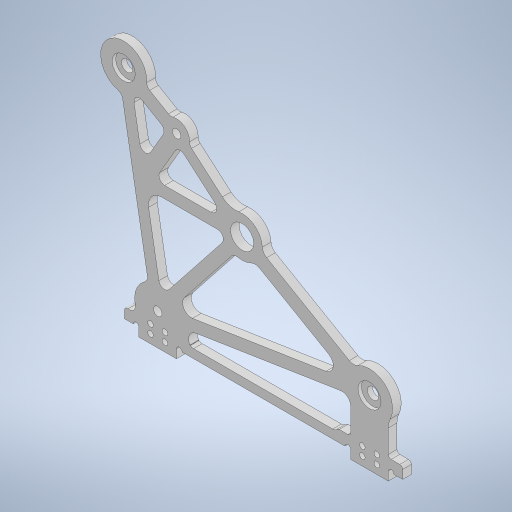
# Autodesk Inventor part: 左フレーム
Saved by Autodesk Inventor 2023 (Build 270158000, 158)
## iProperties
Created: 2022-05-09
Part Number: 左フレーム
Material: 一般
Document SubType Name: Modeling
Designer: muzho
Density: 1 g/cm^3
Appearance: 既定
Author: muzho
Autodesk Inventor part; units mm, degrees
ref_plane "YZ Plane" through (0, 0, 0) normal (1, 0, 0) x (0, 1, 0)
ref_plane "XZ Plane" through (0, 0, 0) normal (0, 1, 0) x (-1, 0, 0)
ref_plane "XY Plane" through (0, 0, 0) normal (0, 0, 1) x (1, 0, 0)
sketch "スケッチ1" plane through (0, 0, 0) normal (0, 0, 1) x (1, 0, 0)
  circle A0 centre (96.1264, 13.4764) radius 8
  circle A1 centre (96.1264, 13.4764) radius 4
  circle A2 centre (11.0035, 69.2097) radius 8
  circle A3 centre (52, 38.9528) radius 37.9528 construction
  circle A4 centre (22.7682, 2) radius 1.5
  circle A5 centre (112.1264, -3) radius 3
  circle A6 centre (112.1264, -3) radius 1.5
  circle A7 centre (74.5, -6) radius 1
  circle A8 centre (69.5, -6) radius 1
  circle A9 centre (69.5, -3) radius 1
  circle A10 centre (74.5, -3) radius 1
  circle A11 centre (64.5, -6) radius 1
  circle A12 centre (79.5, -6) radius 1
  line L0 (65.5, -6) -> (65.5, -9)
  line L1 (65.5, -9) -> (72, -9)
  line L2 (78.5, -9) -> (72, -9)
  line L3 (78.5, -6) -> (78.5, -9)
  circle A13 centre (-14.8489, -6) radius 1
  line L4 (-13.8489, -6) -> (-13.8489, -9)
  line L5 (-13.8489, -9) -> (-7.3489, -9)
  line L6 (-0.8489, -9) -> (-7.3489, -9)
  circle A14 centre (0.1511, -6) radius 1
  circle A15 centre (-4.8489, -6) radius 1
  circle A16 centre (-9.8489, -6) radius 1
  line L7 (-10.8489, -3) -> (-10.8489, -6)
  circle A17 centre (-9.8489, -3) radius 1
  circle A18 centre (-4.8489, -3) radius 1
  line L8 (-3.8489, -3) -> (-3.8489, -6)
  line L9 (-0.8489, -6) -> (-0.8489, -9)
  circle A19 centre (52, 38.9528) radius 4.025
  circle A20 centre (52, 38.9528) radius 7.025
  circle A21 centre (29.2901, 58.5554) radius 1.5
  circle A22 centre (29.2901, 58.5554) radius 4.5
  circle A23 centre (11.0035, 69.2097) radius 2
  line L10 (29.2901, 58.5554) -> (52, 38.9528) construction
  line L11 (31.8618, 53.6936) -> (42.5512, 44.4668)
  arc A24 (33.7847, 58.334) -> (34.4754, 56.7216) centre (35.7823, 58.2356) ccw
  line L12 (34.4754, 56.7216) -> (45.1648, 47.4948)
  line L13 (17.4612, 62.5539) -> (23.9789, 58.7565)
  line L14 (11.0035, 69.2097) -> (29.2901, 58.5554) construction
  line L15 (19.9782, 66.8741) -> (26.496, 63.0767)
  arc A25 (26.496, 63.0767) -> (28.0527, 62.8819) centre (27.5028, 64.8048) ccw
  line L16 (-4.8489, -3) -> (34.2185, -3) construction
  arc A26 (10.6138, 59.8369) -> (9.1157, 61.4356) centre (8.6437, 59.4921) ccw
  arc A27 (30.5306, 0.0647) -> (15.0058, 0.0647) centre (22.7682, 2) ccw
  arc A28 (18.3519, 8.6706) -> (19.2179, 10.683) centre (17.2479, 10.3382) ccw
  line L17 (19.2179, 10.683) -> (10.6138, 59.8369)
  line L18 (11.0035, 69.2097) -> (22.7682, 2) construction
  line L19 (23.158, 11.3727) -> (14.5539, 60.5266)
  circle A29 centre (20.2682, -3) radius 1
  circle A30 centre (20.2682, -6) radius 1
  line L20 (-4.8489, -6) -> (69.5, -6) construction
  line L21 (19.2682, -3) -> (19.2682, -6)
  line L22 (22.7682, 2) -> (22.7682, -10.8027) construction
  circle A31 centre (15.2682, -6) radius 1
  line L23 (16.2682, -6) -> (16.2682, -9)
  line L24 (16.2682, -9) -> (22.7682, -9)
  circle A32 centre (25.2682, -3) radius 1
  line L25 (26.2682, -3) -> (26.2682, -6)
  circle A33 centre (25.2682, -6) radius 1
  circle A34 centre (30.2682, -6) radius 1
  line L26 (29.2682, -6) -> (29.2682, -9)
  line L27 (29.2682, -9) -> (22.7682, -9)
  arc A35 (12.5339, -2.3472) -> (15.0058, 0.0647) centre (13.0652, -0.4191) ccw
  arc A36 (18.1007, -3.1756) -> (11.2685, -5.953) centre (15.2682, -6) ccw construction
  arc A37 (12.5339, -2.3472) -> (11.2682, -3.3113) centre (12.2682, -3.3113) ccw
  line L28 (11.2682, -3.3113) -> (11.2682, -6)
  line L29 (11.2682, -6) -> (14.2682, -6)
  arc A38 (30.5306, 0.0647) -> (33.0026, -2.3472) centre (32.4712, -0.4191) ccw
  arc A39 (34.2682, -3.3113) -> (33.0026, -2.3472) centre (33.2682, -3.3113) ccw
  line L30 (34.2682, -3.3113) -> (34.2682, -6)
  line L31 (34.2682, -6) -> (31.2682, -6)
  arc A40 (24.7001, 56.0216) -> (23.9789, 58.7565) centre (22.9721, 57.0284) ccw
  arc A41 (16.5609, 49.061) -> (20.259, 48.399) centre (18.5309, 49.4058) ccw
  line L32 (20.259, 48.399) -> (24.7001, 56.0216)
  line L33 (29.2901, 58.5554) -> (18.2237, 39.5614) construction
  line L34 (28.8268, 53.1865) -> (19.2074, 36.6759)
  arc A42 (19.2074, 36.6759) -> (18.9654, 35.3243) centre (20.9355, 35.6691) ccw
  arc A43 (31.8618, 53.6936) -> (28.8268, 53.1865) centre (30.5549, 52.1796) ccw
  line L35 (52, 38.9528) -> (22.7682, 2) construction
  line L36 (45.077, 33.712) -> (26.6966, 10.4768)
  arc A44 (23.451, 43.9596) -> (25.1791, 40.9528) centre (25.1791, 42.9528) ccw
  arc A45 (41.2443, 40.9528) -> (42.5512, 44.4668) centre (41.2443, 42.9528) ccw
  line L37 (25.1791, 40.9528) -> (41.2443, 40.9528)
  line L38 (52, 38.9528) -> (21.2682, 38.9528) construction
  arc A46 (45.1648, 47.4948) -> (50.8667, 45.8858) centre (49.7377, 52.7925) ccw
  arc A47 (45.077, 33.712) -> (43.5084, 36.9528) centre (43.5084, 34.9528) ccw
  line L39 (43.5084, 36.9528) -> (24.1067, 36.9528)
  arc A48 (24.1067, 36.9528) -> (19.616, 31.6077) centre (24.1067, 32.3938) ccw
  line L40 (96.1264, 13.4764) -> (96.1264, -6.671) construction
  line L41 (74.5, -3) -> (105.0338, -3) construction
  line L42 (74.5, -6) -> (105.6943, -6) construction
  circle A49 centre (93.6264, -3) radius 1
  circle A50 centre (93.6264, -6) radius 1
  line L43 (92.6264, -3) -> (92.6264, -6)
  circle A51 centre (88.6264, -6) radius 1
  line L44 (89.6264, -6) -> (89.6264, -9)
  line L45 (89.6264, -9) -> (96.1264, -9)
  line L46 (87.6264, -6) -> (84.6264, -6)
  line L47 (84.6264, -6) -> (84.6264, -3)
  arc A52 (85.6264, -2) -> (84.6264, -3) centre (85.6264, -3) ccw
  line L48 (85.6264, -2) -> (88.6264, -2)
  arc A53 (90.3583, -2.3944) -> (86.7859, -2.4486) centre (88.6264, -6) ccw construction
  arc A54 (95.7232, 0.4064) -> (89.7681, -4.0552) centre (93.6264, -3) ccw construction
  arc A55 (88.6264, -2) -> (89.6264, -1) centre (88.6264, -1) ccw
  line L49 (89.6264, -1) -> (89.6264, 6.9294)
  line L50 (102.6264, -1) -> (102.6264, 6.9294)
  arc A56 (103.3284, 9.9934) -> (102.6264, 6.9294) centre (109.6643, 6.9294) ccw
  line L51 (106.6264, -2) -> (103.6264, -2)
  arc A57 (102.6264, -1) -> (103.6264, -2) centre (103.6264, -1) ccw
  arc A58 (107.6264, -3) -> (106.6264, -2) centre (106.6264, -3) ccw
  line L52 (107.6264, -6) -> (107.6264, -3)
  circle A59 centre (103.6264, -6) radius 1
  line L53 (102.6264, -6) -> (102.6264, -9)
  line L54 (102.6264, -9) -> (96.1264, -9)
  circle A60 centre (98.6264, -6) radius 1
  line L55 (99.6264, -3) -> (99.6264, -6)
  circle A61 centre (98.6264, -3) radius 1
  line L56 (104.6264, -6) -> (107.6264, -6)
  line L57 (34.2682, -6) -> (84.6264, -6)
  arc A62 (33.9058, -2.5408) -> (35.1808, -3) centre (35.1808, -1) ccw
  line L58 (34.2185, -3) -> (69.5, -3) construction
  arc A63 (83.3903, -3) -> (84.8811, -2.3333) centre (83.3903, -1) ccw
  line L59 (35.1808, -3) -> (83.3903, -3)
  arc A64 (58.0086, 32.5969) -> (55.1594, 32.6784) centre (56.5086, 29.9989) ccw
  line L60 (58.0086, 32.5969) -> (82.0748, 18.7023)
  line L61 (52, 38.9528) -> (96.1264, 13.4764) construction
  arc A65 (59.0135, 39.3539) -> (60.5086, 36.9271) centre (62.0086, 39.5252) ccw
  line L62 (60.5086, 36.9271) -> (89.1264, 20.4046)
  arc A66 (89.1264, 20.4046) -> (92.1264, 20.4046) centre (90.6264, 23.0027) ccw
  arc A67 (81.0385, 13.1403) -> (82.0748, 18.7023) centre (80.5748, 16.1043) ccw
  arc A68 (89.6264, 6.9294) -> (86.1627, 9.8933) centre (86.6264, 6.9294) ccw
  line L63 (81.0385, 13.1403) -> (34.8172, 5.9093)
  line L64 (86.1627, 9.8933) -> (36.0087, 2.0471)
  line L65 (96.1264, 13.4764) -> (22.7682, 2) construction
  line L66 (48.3565, 31.4104) -> (32.0007, 10.7345)
  arc A69 (50.3849, 32.116) -> (48.3565, 31.4104) centre (49.9251, 30.1696) ccw
  arc A70 (32.0007, 10.7345) -> (34.8172, 5.9093) centre (34.3535, 8.8733) ccw
  arc A71 (36.0087, 2.0471) -> (34.0693, -2.7127) centre (36.4724, -0.9169) ccw
  circle A72 centre (11.0035, 69.2097) radius 4
  arc A73 (17.4612, 62.5539) -> (14.5539, 60.5266) centre (16.4777, 60.866) ccw
  arc A74 (18.9888, 68.7237) -> (19.9782, 66.8741) centre (20.9851, 68.6022) ccw
  arc A75 (23.158, 11.3727) -> (26.6966, 10.4768) centre (25.128, 11.7176) ccw
  circle A76 centre (96.1264, 13.4764) radius 2
  point P0 (0, 0)
  point P1 (33.9975, -2.6124)
  point P2 (28.0527, 62.8819)
  point P3 (31.2682, -6)
  dimension "d191" = 2
  dimension "d192" = 2
  dimension "d212" = 2
  dimension "d213" = 2
  dimension "d180" = 8.05
  dimension "d181" = 3
  dimension "d182" = 3
  dimension "d183" = 3
  dimension "d184" = 4
  dimension "d185" = 2
  dimension "d186" = 2.5
  dimension "d187" = 2
  dimension "d188" = 16
  dimension "d189" = 2
  dimension "d190" = 2
  dimension "d193" = 2
  dimension "d194" = 5
  dimension "d195" = 3
  dimension "d196" = 2.5
  dimension "d197" = 2
  dimension "d198" = 3
  dimension "d199" = 1
  dimension "d200" = 3
  dimension "d201" = 2
  dimension "d202" = 2
  dimension "d203" = 2
  dimension "d204" = 2
  dimension "d205" = 2
  dimension "d206" = 2
  dimension "d207" = 2
  dimension "d208" = 2
  dimension "d209" = 2
  dimension "d210" = 2
  dimension "d211" = 2
  dimension "d214" = 2
  dimension "d215" = 5
  dimension "d216" = 2.5
  dimension "d217" = 3
  dimension "d218" = 3
  dimension "d219" = 1
  dimension "d220" = 3
  dimension "d221" = 3
  dimension "d222" = 1
  dimension "d223" = 2
  dimension "d224" = 2
  dimension "d225" = 3
  dimension "d226" = 3
  dimension "d227" = 3
  dimension "d228" = 5
  dimension "d229" = 2.5
  dimension "d230" = 3
  dimension "d231" = 3
  dimension "d232" = 4
  dimension "d233" = 2
  dimension "d234" = 2
  dimension "d235" = 4
  dimension "d236" = 3
  dimension "d237" = 3
  dimension "d238" = 8
  dimension "d239" = 2
  dimension "d242" = 4
  constraints: 134 end point, 96 point on circle, 67 tangent, 59 centre point, 36 symmetric about line, 22 point on line, 19 vertical, 16 horizontal, 16 horizontal alignment, 11 parallel, 7 coincident, 6 perpendicular, 2 concentric, 53 other
  measures "d180" diameter of A19
  measures "d181" radial gap between concentric circles of A19 A20
  measures "d182" diameter of A21
  measures "d183" radial gap between concentric circles of A21 A22
  measures "d184" diameter of A23
  measures "d185" distance between parallel lines of L11 L10
  measures "d186" distance between parallel lines of L13 L14
  measures "d187" radius of A26
  measures "d188" diameter of A27
  measures "d189" radius of A28
  measures "d190" distance between parallel lines of L17 L18
  measures "d193" diameter of A31
  measures "d194" distance of point (20.268, -6) A31.centre
  measures "d195" distance of L23.start L23.end
  measures "d196" distance from line of L22 point (20.268, -3)
  measures "d197" radius of A35
  measures "d198" radial gap between concentric circles of A31 A36
  measures "d199" radius of A37
  measures "d200" distance of L28.end L29.end
  measures "d201" radius of A25
  measures "d202" radius of A41
  measures "d203" radius of A40
  measures "d204" radius of A42
  measures "d205" radius of A43
  measures "d206" radius of A24
  measures "d207" radius of A44
  measures "d208" distance between parallel lines of L38 L37
  measures "d209" radius of A45
  measures "d210" radius of A47
  measures "d211" distance between parallel lines of L39 L38
  measures "d214" diameter of A51
  measures "d215" distance of A51.centre point (93.626, -6)
  measures "d216" distance from line of L40 point (93.626, -3)
  measures "d217" distance of L44.start L44.end
  measures "d218" distance of L46.start L46.end
  measures "d219" radius of A52
  measures "d220" radial gap between concentric circles of A51 A53
  measures "d222" radius of A55
  measures "d223" radius of A62
  measures "d224" radius of A63
  measures "d225" radius of A64
  measures "d226" radius of A65
  measures "d227" radius of A66
  measures "d228" distance between parallel lines of L60 L62
  measures "d229" distance between parallel lines of L62 L61
  measures "d230" radius of A67
  measures "d231" radius of A68
  measures "d232" distance between parallel lines of L64 L63
  measures "d233" distance between parallel lines of L64 L65
  measures "d234" radius of A69
  measures "d235" distance between parallel lines of L36 L66
  measures "d236" radius of A70
  measures "d237" radius of A71
  measures "d238" diameter of A72
  measures "d239" radius of A74
  measures "d242" diameter of A76
extrude "押し出し1" add sketch "スケッチ1" along normal blind 3 contours A0 | A0 A56 L50 A57 L51 A58 L52 L56 A59 L53 L54 L45 L44 A51 L46 L47 A52 L48 A55 L49 A68 L64 A71 A62 A39 A38 A27 A75 L36 A47 L39 A48 L19 A42 L34 A44 L37 A45 L11 A43 A22 A24 L12 A46 A20 A69 L66 A70 L63 A67 L60 A64 A65 L62 A66 | A20 | A22 | A43 L34 A42 L19 A41 L32 A40 A22 | A22 A40 L13 A73 L19 A75 A27 A28 L17 A26 A2 A74 L15 A25 | A2 | L57 A12 A7 A8 A11 L30 A39 A71 A62 L59 A9 A10 A63 A52 L47 | A27 A38 A39 L30 L31 A34 L26 L27 L24 L23 A31 L29 L28 A37 A35 | L57 A12 | L57 A7 | A10 L59 | L57 A8 | A9 L59 | L57 A11 picked at (79.7495, -5.6194) picked at (74.7495, -5.6194) picked at (74.2505, -3.3806) picked at (69.7495, -5.6194) picked at (69.2505, -3.3806) picked at (64.7495, -5.6194)
extrude "押し出し2" add sketch "スケッチ1" along normal blind 1.8 contours A1 | A72
equation "\"d229\" = 0.5 * d228"
equation "\"d233\" = 0.5 * d232"
